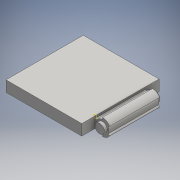
# Autodesk Inventor part: ThreeEdge
Saved by Autodesk Inventor 2016 (Build 200138000, 138)
## iProperties
Created: 2016-10-09
Part Number: ThreeEdge
Material: Generic
Document SubType Name: Modeling
Designer: Kevin
Density: 1 g/cm^3
Appearance: Default
Author: Kevin
Autodesk Inventor part; units mm, degrees
ref_plane "YZ Plane" through (0, 0, 0) normal (1, 0, 0) x (0, 1, 0)
ref_plane "XZ Plane" through (0, 0, 0) normal (0, 1, 0) x (-1, 0, 0)
ref_plane "XY Plane" through (0, 0, 0) normal (0, 0, 1) x (1, 0, 0)
sketch "Sketch1" plane through (0, 0, 0) normal (0, 0, 1) x (1, 0, 0)
  line L0 (0, 0) -> (530.86, 0)
  line L1 (530.86, 0) -> (530.86, -541.02)
  line L2 (530.86, -541.02) -> (0, -541.02)
  line L3 (0, -541.02) -> (0, 0)
  dimension "d0" = 530.86
  dimension "d1" = 541.02
  constraints: 8 end point, 2 parallel, 1 horizontal, 1 perpendicular
  measures "d0" distance of L1.end L2.end
  measures "d1" distance of L0.end L1.end
extrude "Extrusion1" add sketch "Sketch1" along normal blind 76.2
ref_plane "Work Plane1" through (530.86, -450.59, 76.2) normal (0, -1, 0) x (1, 0, 0)
sketch "Sketch5" plane through (530.86, -450.59, 76.2) normal (0, -1, 0) x (1, 0, 0)
  line L0 (0, -76.2) -> (0, 0) projected
  line L1 (0, -76.2) -> (0, -38.1)
  circle A0 centre (55, -38.1) radius 45
  arc A1 (87.454, -69.2727) -> (100, -38.1) centre (55, -38.1) ccw
  arc A2 (87.454, -69.2727) -> (99.1479, -29.3843) centre (55, -38.1) ccw
  arc A3 (52.3903, 6.8243) -> (19.4107, -10.5609) centre (55, -38.1) ccw
  arc A4 (104.7965, -9.35) -> (55, 19.4) centre (55, -38.1) ccw
  arc A5 (55, -95.6) -> (104.7965, -66.85) centre (55, -38.1) ccw
  arc A6 (5.2035, -9.35) -> (5.2035, -66.85) centre (55, -38.1) ccw
  line L2 (5.2035, -9.35) -> (16.0289, -15.6)
  line L3 (55, 19.4) -> (55, 6.9)
  line L4 (104.7965, -9.35) -> (93.9711, -15.6)
  line L5 (104.7965, -66.85) -> (93.9711, -60.6)
  line L6 (55, -95.6) -> (55, -83.1)
  line L7 (5.2035, -66.85) -> (16.0289, -60.6)
  point P0 (-530.86, -76.2)
  dimension "d13" = 38.1
  constraints: 14 end point, 14 point on circle, 6 centre point, 2 concentric, 1 midpoint, 14 other
  measures "d13" distance of L0.start L1.end
extrude "Extrusion7" add sketch "Sketch5" against normal blind 350
sketch "Sketch8" plane through (530.86, -450.59, 76.2) normal (0, -1, 0) x (1, 0, 0)
  line L0 (0, -54.8705) -> (0, -21.3295) projected
  line L1 (0, -38.1) -> (55, -38.1)
  circle A0 centre (55, -38.1) radius 32.5
  point P0 (-530.86, -76.2)
  dimension "d28" = 55
  dimension "d29" = 65
  constraints: 2 end point, 1 centre point, 1 coincident, 1 horizontal, 1 midpoint
  measures "d28" distance of L1.start L1.end
  measures "d29" diameter of A0
extrude "Extrusion8" add sketch "Sketch8" along normal blind 20
sketch "Sketch9" plane through (530.86, -100.59, 76.2) normal (0, 1, 0) x (1, 0, 0)
  line L0 (0, 54.8705) -> (0, 21.3295) projected
  line L1 (0, 38.1) -> (55, 38.1)
  circle A0 centre (55, 38.1) radius 32.5
  point P0 (-530.86, 76.2)
  dimension "d32" = 55
  constraints: 2 end point, 1 centre point, 1 coincident, 1 horizontal, 1 midpoint
  measures "d32" distance of L1.start L1.end
extrude "Extrusion9" add sketch "Sketch9" along normal blind 20
body "Solid1"
